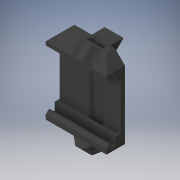
# Autodesk Inventor part: extruder_breakout_mount
Saved by Autodesk Inventor 2017 (Build 210142000, 142)
## iProperties
Created: 2017-06-16
Part Number: extruder_breakout_mount
Material: Generic
Document SubType Name: Modeling
Designer: yibre
Density: 1 g/cm^3
Appearance: Default
Author: yibre
Autodesk Inventor part; units mm, degrees
ref_plane "Work Plane1" through (2, -31.725, -1.9) normal (1, 0, 0) x (0, 0, -1)
sketch "Sketch2" plane through (2, -31.725, -1.9) normal (1, 0, 0) x (0, 0, -1)
  line L0 (-6, 6.0325) -> (-7.5515, 6.0325) construction
  line L1 (-6, 29.4005) -> (-7.5515, 29.4005) construction
  line L2 (-7.5515, 29.4005) -> (-7.5515, 6.0325) construction
  line L3 (-6, 6.0325) -> (-6, 29.4005) construction
  line L4 (-7.7515, 5.4325) -> (-5.8, 5.4325)
  line L5 (-5.8, 5.4325) -> (-5.8, 30.0005)
  line L6 (-5.8, 30.0005) -> (-7.7515, 30.0005)
  line L7 (-7.7515, 30.0005) -> (-7.7515, 5.4325)
  line L8 (3.2015, 0.1) -> (-1.9, 5.2015) projected
  line L9 (-1.9, 6) -> (-1.9, 29) projected
  line L10 (-1.9, 5.2015) -> (-1.9, 6) projected
  line L11 (3.2015, 34.9) -> (-9.2515, 34.9)
  line L12 (-9.2515, 34.9) -> (-9.2515, 0.1)
  line L13 (-9.2515, 0.1) -> (3.2015, 0.1)
  line L14 (-1.9, 29.7985) -> (3.2015, 34.9)
  line L15 (-1.9, 29) -> (-1.9, 29.7985)
  dimension "d7" = 0.6
  dimension "d8" = 0.6
  dimension "d9" = 0.2
  dimension "d10" = 0.2
  dimension "d11" = 1.5
  constraints: 22 end point, 3 parallel, 3 perpendicular, 2 horizontal, 2 vertical, 4 other
  measures "d7" distance between parallel lines of L1 L6
  measures "d8" distance between parallel lines of L4 L0
  measures "d9" distance between parallel lines of L7 L2
  measures "d10" distance between parallel lines of L5 L3
  measures "d11" distance between parallel lines of L12 L7
ref_plane "Work Plane3" through (11, -31.725, -5.9) normal (-1, 0, 0) x (0, 0, 1)
extrude "Extrusion2" add sketch "Sketch2" along normal up to surface (9 mm away)
sketch "Sketch3" plane through (2, -31.725, -1.9) normal (-1, 0, 0) x (0, 0, 1)
  line L0 (7.7515, 30.0005) -> (7.7515, 5.4325) projected
  line L1 (7.7515, 5.4325) -> (5.8, 5.4325) projected
  line L2 (5.8, 5.4325) -> (5.8, 30.0005) projected
  line L3 (5.8, 30.0005) -> (7.7515, 30.0005) projected
  line L4 (-3.2015, 0.1) -> (1.9, 5.2015) construction
  line L5 (9.2515, 0.1) -> (-3.2015, 0.1) projected
  line L6 (9.2515, 34.9) -> (9.2515, 0.1) projected
  line L7 (-3.2015, 34.9) -> (9.2515, 34.9) projected
  line L8 (2, 2) -> (2, 33) projected
  line L9 (2, 33) -> (2, 34.9)
  line L10 (2, 2) -> (2, 0.1)
  line L11 (1.9, 29.7985) -> (-3.2015, 34.9) projected
  line L12 (1.9, 5.2015) -> (1.9, 29.7985) projected
  point P0 (1.9, 31.725)
  constraints: 4 end point, 3 point on line, 1 vertical
extrude "Extrusion3" add sketch "Sketch3" along normal blind 10
sketch "Sketch4" plane through (11, -31.625, 7.3515) normal (1, 0, 0) x (0, 0, -1)
  line L0 (1.5, 5.3325) -> (3.4515, 5.3325) projected
  line L1 (3.4515, 5.3325) -> (3.4515, 29.9005) projected
  line L2 (3.4515, 29.9005) -> (1.5, 29.9005) projected
  line L3 (1.5, 29.9005) -> (1.5, 5.3325) projected
  line L4 (7.2515, 0) -> (0, 0) projected
  line L5 (0, 0) -> (0, 34.8) projected
  line L6 (0, 34.8) -> (7.2515, 34.8) projected
  line L7 (7.2515, 34.8) -> (7.2515, 0) projected
  point P0 (7.3515, 31.625)
extrude "Extrusion4" add sketch "Sketch4" along normal blind 5
sketch "Sketch5" plane through (-8, -31.625, 7.3515) normal (0, 0, 1) x (1, 0, 0)
  line L0 (0, 29.9005) -> (24, 29.9005) projected
  line L1 (0, 5.3325) -> (0, 29.9005) projected
  line L2 (0, 5.3325) -> (24, 5.3325) projected
  line L3 (24, 29.9005) -> (24, 5.3325) projected
  line L4 (0, 6.8325) -> (24, 6.8325)
  line L5 (24, 6.8325) -> (24, 28.4005)
  line L6 (24, 28.4005) -> (0, 28.4005)
  line L7 (0, 28.4005) -> (0, 6.8325)
  point P0 (8, 31.625)
  dimension "d18" = 1.5
  dimension "d19" = 1.5
  constraints: 8 end point, 2 parallel, 2 point on line, 1 horizontal, 1 perpendicular
  measures "d18" distance between parallel lines of L0 L6
  measures "d19" distance between parallel lines of L2 L4
extrude "Extrusion5" cut sketch "Sketch5" against normal up to next contours L6 L3 L4 L1
chamfer "Chamfer1" distance 1 angle 45 2 edges at (4, -3.2245, 7.3515) (4, -24.7925, 7.3515)
chamfer "Chamfer2" distance 4 angle 45 6 edges at (4, 3.175, 7.3515) (4, -31.625, 7.3515) (-8, -31.625, 3.7257) (-8, 3.175, 3.7257) (16, 3.175, 3.7257) (16, -31.625, 3.7257)
sketch "Sketch6" plane through (2, -31.625, -5.1015) normal (0, -1, 0) x (1, 0, 0)
  line L0 (1.5, 7.6015) -> (7.5, 7.6015)
  line L1 (7.5, 7.6015) -> (7.5, 6.1015)
  line L2 (7.5, 6.1015) -> (1.5, 6.1015)
  line L3 (1.5, 6.1015) -> (1.5, 7.6015)
  line L4 (0, 0) -> (9, 0) projected
  line L5 (4.4809, 14.182) -> (4.4809, 20.278) projected
  line L6 (4.5, 6.1015) -> (4.5, 0)
  point P0 (-2, 5.1015)
  point P1 (0, 5.1015)
  dimension "d28" = 6
  dimension "d29" = 1.5
  dimension "d53" = 1
  constraints: 10 end point, 2 midpoint, 2 parallel, 2 perpendicular, 1 horizontal
  measures "d28" distance of L1.end L2.end
  measures "d29" distance of L0.end L1.end
  measures "d53" distance from line of L2 point (0, 5.102)
extrude "Extrusion6" cut sketch "Sketch6" against normal through all
fillet "Fillet1" radius 2 2 edges at (6.5, -31.625, 1) (6.5, 3.175, 1)
sketch "Sketch7" plane through (16, -31.625, 7.3515) normal (1, 0, 0) x (0, 0, -1)
  line L0 (3.4515, 29.9005) -> (3.4515, 5.3325) projected
  line L1 (3.4515, 26.9005) -> (5.4515, 26.9005)
  line L2 (5.4515, 26.9005) -> (5.4515, 8.3325)
  line L3 (5.4515, 8.3325) -> (3.4515, 8.3325)
  line L4 (3.4515, 8.3325) -> (3.4515, 26.9005)
  line L5 (3.4515, 5.3325) -> (1.5, 5.3325) projected
  line L6 (1.5, 29.9005) -> (3.4515, 29.9005) projected
  point P0 (7.3515, 31.625)
  dimension "d34" = 3
  dimension "d35" = 3
  dimension "d36" = 2
  constraints: 8 end point, 2 parallel, 1 horizontal, 1 perpendicular, 1 point on line
  measures "d34" distance between parallel lines of L5 L3
  measures "d35" distance between parallel lines of L6 L1
  measures "d36" distance of L2.end L3.end
extrude "Extrusion7" cut sketch "Sketch7" against normal through all
move faces "Move1" translate (-0.8, 0, 0) faces at (11, -29.9245, -1.6672)
move faces "Move2" translate (0.8, 0, 0) faces at (2, -29.9245, -1.6672)
ref_plane "Work Plane4" through (6.5, -26.5235, 0) normal (-1, 0, 0) x (0, 0, 1)
sketch "Sketch8" plane through (6.5, -26.5235, 0) normal (-1, 0, 0) x (0, 0, 1)
  line L0 (7.3515, 25.6985) -> (3.3515, 29.6985) projected
  line L1 (6.5889, 26.461) -> (4.114, 28.9359)
  line L2 (4.114, 28.9359) -> (4.9979, 29.8198)
  line L3 (4.9979, 29.8198) -> (7.4728, 27.3449)
  line L4 (7.4728, 27.3449) -> (6.5889, 26.461)
  line L5 (7.3515, 25.6985) -> (8.9425, 27.2895)
  line L6 (8.9425, 27.2895) -> (4.9425, 31.2895)
  line L7 (4.9425, 31.2895) -> (3.3515, 29.6985)
  point P0 (0, 26.5235)
  point P1 (5.3515, 27.6985)
  dimension "d45" = 3.5
  dimension "d46" = 1.25
  dimension "d47" = 1
  constraints: 14 end point, 3 perpendicular, 2 midpoint, 2 parallel, 2 point on line
  measures "d45" distance of L1.start L1.end
  measures "d46" distance of L1.end L2.end
  measures "d47" distance between parallel lines of L6 L3
extrude "Extrusion8" add sketch "Sketch8" along normal mid plane 7 contours L0 L4 L3 L2 L7 L6 L5
ref_plane "Work Plane5" through (-8, -14.225, 20.7515) normal (0, 1, 0) x (-1, 0, 0)
mirror "Mirror1" about plane through (-8, -14.225, 20.7515) normal (0, 1, 0) of "Extrusion8"
chamfer "Chamfer3" distance 1 angle 45 6 edges at (3.5, -31.0392, 0.4142) (3.5, -14.225, 1) (3.5, 2.5892, 0.4142) (9.5, -31.0392, 0.4142) (9.5, -14.225, 1) (9.5, 2.5892, 0.4142)
chamfer "Chamfer4" distance 2.25 angle 45 4 edges at (3, -31.216, 6.9425) (10, -31.216, 6.9425) (3, 2.766, 6.9425) (10, 2.766, 6.9425)
sketch "Sketch9" plane through (16, -31.625, 7.3515) normal (1, 0, 0) x (0, 0, -1)
  line L0 (1.5, 29.9005) -> (3.4515, 29.9005) projected
  line L1 (3.4515, 5.3325) -> (1.5, 5.3325) projected
  line L2 (2.4757, 29.9005) -> (2.4757, 5.3325)
  line L3 (2.4757, 3.8325) -> (2.4757, 31.4005) construction
  line L4 (2.7257, 3.8325) -> (2.7257, 31.4005)
  line L5 (2.2257, 31.4005) -> (2.2257, 3.8325)
  arc A0 (2.2257, 3.8325) -> (2.7257, 3.8325) centre (2.4757, 3.8325) ccw
  arc A1 (2.7257, 31.4005) -> (2.2257, 31.4005) centre (2.4757, 31.4005) ccw
  point P0 (7.3515, 31.625)
  point P1 (2.4757, 17.6165)
  dimension "d60" = 0.5
  dimension "d61" = 1.5
  constraints: 10 end point, 5 midpoint, 4 point on circle, 4 tangent, 2 centre point, 1 parallel, 1 point on line
  measures "d60" diameter of A1
  measures "d61" distance from line of L0 L3.end
extrude "Extrusion9" cut sketch "Sketch9" against normal through all
body "Solid2"
